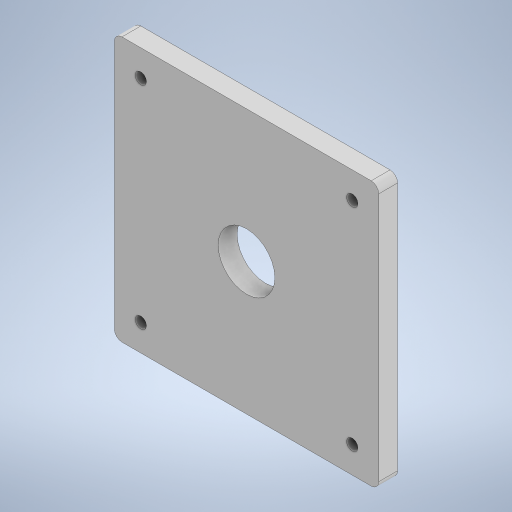
# Autodesk Inventor part: Motor clamp p1
Saved by Autodesk Inventor 2023 (Build 270158000, 158)
## iProperties
Created: 2022-06-04
Part Number: Motor clamp p1
Material: Generic
Document SubType Name: Modeling
Designer: prana_p9lsmih
Density: 1 g/cm^3
Appearance: Default
Author: prana_p9lsmih
Autodesk Inventor part; units mm, degrees
ref_plane "YZ Plane" through (0, 0, 0) normal (1, 0, 0) x (0, 1, 0)
ref_plane "XZ Plane" through (0, 0, 0) normal (0, 1, 0) x (-1, 0, 0)
ref_plane "XY Plane" through (0, 0, 0) normal (0, 0, 1) x (1, 0, 0)
sketch "Sketch1" plane through (0, 0, 0) normal (0, 0, 1) x (1, 0, 0)
  line L0 (0, 0) -> (70, 0)
  line L1 (70, 0) -> (70, 70)
  line L2 (70, 70) -> (0, 70)
  line L3 (0, 70) -> (0, 0)
  dimension "d0" = 70
  dimension "d1" = 70
  constraints: 8 end point, 3 perpendicular, 1 horizontal
  measures "d0" distance of L0.start L0.end
  measures "d1" distance of L0.end L1.end
extrude "Extrusion1" add sketch "Sketch1" along normal blind 5
sketch "Sketch2" plane through (0, 0, 5) normal (0, 0, 1) x (1, 0, 0)
  line L0 (70, 70) -> (0, 70) projected
  line L1 (70, 0) -> (70, 70) projected
  point P0 (0, 0)
  point P1 (35, 35)
  dimension "d4" = 35
  dimension "d5" = 35
  measures "d4" distance from line of L0 point (35, 35)
  measures "d5" distance from line of L1 point (35, 35)
hole "Hole1" at (35, 35, 5) direction (0, 0, -1) diameter 15 end through all
fillet "Fillet1" radius 2 4 edges at (70, 70, 2.5) (70, 0, 2.5) (0, 0, 2.5) (0, 70, 2.5)
sketch "Sketch3" plane through (0, 0, 5) normal (0, 0, 1) x (1, 0, 0)
  line L0 (2, 0) -> (68, 0) projected
  line L1 (70, 2) -> (70, 68) projected
  point P0 (0, 0)
  point P1 (63, 7)
  dimension "d14" = 7
  dimension "d15" = 7
  measures "d14" distance from line of L0 point (63, 7)
  measures "d15" distance from line of L1 point (63, 7)
hole "Hole2" at (63, 7, 5) direction (0, 0, -1) diameter 3 end through all
sketch "Sketch4" plane through (0, 0, 5) normal (0, 0, 1) x (1, 0, 0)
  line L0 (2, 0) -> (68, 0) projected
  line L1 (0, 68) -> (0, 2) projected
  line L2 (68, 70) -> (2, 70) projected
  line L3 (70, 2) -> (70, 68) projected
  point P0 (0, 0)
  point P1 (7, 7)
  point P2 (7, 63)
  point P3 (63, 63)
  dimension "d23" = 7
  dimension "d24" = 7
  dimension "d25" = 7
  dimension "d26" = 7
  dimension "d27" = 7
  dimension "d28" = 7
  measures "d23" distance from line of L0 point (7, 7)
  measures "d24" distance from line of L1 point (7, 7)
  measures "d25" distance from line of L1 point (7, 63)
  measures "d26" distance from line of L2 point (7, 63)
  measures "d27" distance from line of L2 point (63, 63)
  measures "d28" distance from line of L3 point (63, 63)
hole "Hole3" at (7, 7, 5) at (7, 63, 5) at (63, 63, 5) direction (0, 0, -1) diameter 3 end through all
body "Solid1"
